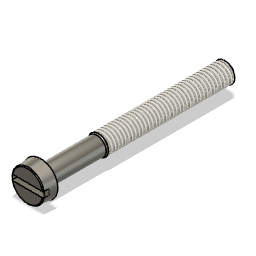
Drill_Jig_Assembly (Autodesk Fusion 360 archive; units mm, degrees)
design "Cheese Head Screw ISO 1207 - M6 x 55 Steel 10.9 Plain"
description: Cheese Head Screw ISO 1207 - M6 x 55
Autodesk Fusion 360 part; units mm, degrees
sketch "Sketch1" plane through (0, 0, 0) normal (0, 1, 0) x (1, 0, 0)
  line L0 (-3, 55) -> (0, 55)
  line L1 (0, 55) -> (0, -3.9)
  line L2 (-2.6932, 0) -> (-5, 0)
  line L3 (0, -3.9) -> (-4.4297, -3.9)
  line L4 (-4.6788, -3.6718) -> (-5, 0)
  arc A0 (-4.6788, -3.6718) -> (-4.4297, -3.9) centre (-4.4297, -3.65) ccw
  line L5 (-2.6932, 0) -> (-2.6932, 16.4687)
  line L6 (-3, 17) -> (-3, 55)
  line L7 (-3, 55) -> (0, 55)
  line L8 (-3, 17) -> (-2.6932, 16.4687)
  line L9 (0, -1.75) -> (0, -22.5)
  dimension "d66" = 10
  dimension "d67" = 3.9
  dimension "d68" = 55
  dimension "d83" = 0.25
  dimension "d93" = 5.3865
  dimension "d95" = 6
  dimension "d97" = 150
  dimension "d98" = 17
  dimension "d100" = 85
  constraint collinear origin L1.end L0.end
  constraint coincident origin L2
  constraint vertical L1
  constraint perpendicular L1 L3
  constraint tangent L3 A0
  constraint tangent L4 A0
  constraint perpendicular L2 L5
  constraint perpendicular L2 L6
  constraint perpendicular L6 L7
  constraint coincident L0.start L6.end
  measures "d67" vertical distance of L1.end L2.end
  measures "d68" distance of origin L0.end
  measures "d83" radius of A0
  measures "d97" angle of L6 L8
  measures "d98" vertical distance of L2.start L6.start
  measures "d100" angle of L2 L4
revolve "Revolve1" add sketch "Sketch1" angle 360 about axis through (0, 0, -55) along (0, 0, 1)
ref_plane "WorkPlane1" through (0, 0, 3.9) normal (0, 0, 1) x (1, 0, 0)
sketch "Sketch7" plane through (0, 0, 3.9) normal (0, 0, 1) x (1, 0, 0)
  line L0 (-4.6788, 0.8) -> (4.6788, 0.8)
  line L1 (4.6788, 0.8) -> (4.6788, -0.8)
  line L2 (4.6788, -0.8) -> (-4.6788, -0.8)
  line L3 (-4.6788, -0.8) -> (-4.6788, 0.8)
  line L4 (-4.6788, 0) -> (4.6788, 0) construction
  circle A0 centre (0, 0) radius 4.6788
  dimension "d77" = 1.6
  constraint horizontal L0
  constraint vertical L1
  constraint horizontal L2
  constraint vertical L3
  constraint midpoint L3 L4.start
  constraint midpoint L1 L4.end
  constraint coincident A0.centre L4
  constraint tangent L3 A0
  constraint tangent L1 A0
  measures "d77" distance of L0.end L1.end
extrude "Extrude3" cut sketch "Sketch7" against normal blind 1.6 contours L0 L2 A0
thread "Thread1" "ISO Metric profile 6.0 M6x1 6g" major diameter 5.884 minor diameter 4.7435 pitch 1 angle 60 resizes the face on face at (-2.9963, 0.1495, -29.6667)
sketch "Sketch8" plane through (0, 0, 0) normal (0, 1, 0) x (1, 0, 0)
  line L0 (0, 55) -> (0, -3.9)
  line L1 (0, 55) -> (-3.06, 55)
  line L2 (-3.06, 55) -> (-3.06, 53.8)
  line L3 (-3.06, 53.8) -> (-1.5, 55)
  dimension "d109" = 1.5
  dimension "d110" = 3.06
  dimension "d111" = 1.2
  constraint coincident L0.start L1.start
  constraint perpendicular L0 L1
  constraint perpendicular L1 L2
  constraint coincident L1 L3.end
  measures "d109" horizontal distance of origin L3.end
  measures "d110" horizontal distance of origin L1.end
  measures "d111" distance of L1.end L2.end
revolve "Revolve3" cut sketch "Sketch8" angle 360 about axis through (0, 0, 1.75) along (0, 0, 1)
equation "adsk_nomlen = 55.00 mm"
equation "adsk_headh = 3.90 mm"
equation "adsk_headdia = 10.00 mm"
equation "adsk_nomdia = 6.00 mm"
equation "d66 = adsk_headdia"
equation "d67 = adsk_headh"
equation "d68 = adsk_nomlen"
equation "d71 = adsk_headh"
equation "adsk_slotdepth = 1.60 mm"
equation "adsk_slotw = 1.60 mm"
equation "d77 = adsk_slotw"
equation "d78 = -adsk_slotdepth"
equation "adsk_thrlen = 38.00 mm"
equation "d83 = adsk_headr"
equation "adsk_headr = 0.25 mm"
equation "d93 = adsk_grpdia"
equation "d95 = adsk_nomdia"
equation "d98 = adsk_nomlen - adsk_thrlen"
equation "adsk_grpdia = 5.3865 mm"
equation "adsk_endpointdia = adsk_nomdia / 2"
equation "adsk_startlen = 0.2 * adsk_nomdia"
equation "d109 = adsk_endpointdia / 2"
equation "d110 = adsk_nomdia * 0.51"
equation "d111 = adsk_startlen"

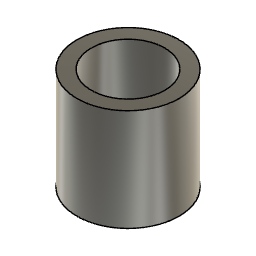
design "Bush case case hardened"
Autodesk Fusion 360 part; units mm, degrees
sketch "Sketch1" plane through (0, 0, 0) normal (0, 1, 0) x (1, 0, 0)
  line L0 (9, -12.5) -> (9, 0)
  line L1 (12.5, 0) -> (12.5, -12.5)
  line L2 (12.5, -12.5) -> (9, -12.5)
  line L3 (12.5, 0) -> (12.5, 12.5)
  line L4 (12.5, 12.5) -> (9, 12.5)
  line L5 (9, 12.5) -> (9, 0)
  line L6 (0, 0) -> (0, -12.5)
  line L7 (0, -12.5) -> (0, 12.5)
  dimension "d3" = 12.5
  constraint perpendicular L0 L2
  constraint coincident L6.start origin
  constraint perpendicular L2 L6
  constraint perpendicular L4 L7
  measures "d3" distance of L6.start L1.start
revolve "Revolve1" add sketch "Sketch1" angle 360 about axis through (0, 0, 12.5) along (0, 0, -1)
equation "d3 = ( 25 / 2 ) * 1 mm"

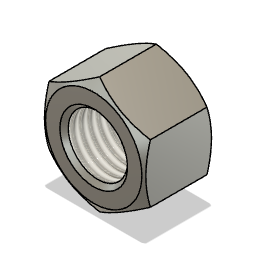
design "Hexagon High Nut ISO 4033 - M20 Steel 6 Plain"
description: Hexagon High Nut ISO 4033 - M20
Autodesk Fusion 360 part; units mm, degrees
sketch "Sketch1" plane through (0, 0, 0) normal (0, 1, 0) x (1, 0, 0)
  line L0 (0, 0.8114) -> (0, -2.1886)
  line L1 (-10, 0) -> (-14.25, 0)
  line L2 (-14.25, 0) -> (-17.325, -1.7754)
  line L3 (-17.325, -1.7754) -> (-17.325, -18.5246)
  line L4 (-17.325, -18.5246) -> (-14.25, -20.3)
  line L5 (-14.25, -20.3) -> (-10, -20.3)
  line L6 (-10, -20.3) -> (-10, 0)
  dimension "d121" = 20
  dimension "d122" = 30
  dimension "d123" = 30
  dimension "d125" = 28.5
  dimension "d126" = 20.3
  dimension "d127" = 28.5
  dimension "d128" = 34.65
  constraint vertical L0
  constraint coincident L0 L0.end
  constraint coincident origin L0
  constraint horizontal L1
  constraint perpendicular L1 L3
  constraint perpendicular L3 L5
  constraint perpendicular L5 L6
  constraint coincident origin L1
  measures "d122" angle of L1 L2
  measures "d123" angle of L4 L5
  measures "d126" distance of L1.start L5.end
revolve "Revolve1" add sketch "Sketch1" angle 360 about axis through (0, 0, -0.8114) along (0, 0, 1)
sketch "Sketch8" plane through (0, 0, 20.3) normal (0, 0, 1) x (1, 0, 0)
  line L0 (0, 0) -> (-30, 0) construction
  line L1 (-15, -8.6692) -> (-15, 8.6692)
  circle A0 centre (0, 0) radius 10
  circle A1 centre (0, 0) radius 17.325
  dimension "d114" = 15
  constraint horizontal L0
  constraint perpendicular L0 L1
  constraint midpoint L0 L1
  constraint coincident L0.start A0.centre
  constraint coincident L1.end A1
  measures "d114" distance of L0.start L1
extrude "Extrude5" cut sketch "Sketch8" against normal blind 20.3 contours L1 A1 picked at (-15.3751, 2.1116)
pattern_circular "C-Pattern2" count 6 over 360 about axis through (0, 0, 1.75) along (0, 0, 1) of "Extrude5"
thread "Thread3" "ISO Metric profile 20.0 M20x2.5 6H" major diameter 20.2925 minor diameter 17.519 pitch 2.5 angle 60 resizes the face on face at (-9.9503, 0.9957, 13.5333)
sketch "Sketch12" plane through (0, 0, 0) normal (0, 1, 0) x (1, 0, 0)
  line L0 (8.7595, -20.3) -> (-8.7595, -20.3)
  line L1 (14.25, -20.3) -> (-14.25, -20.3)
  line L2 (14.25, 0) -> (-14.25, 0)
  line L3 (8.7595, 0) -> (-8.7595, 0)
  line L4 (-10, 0) -> (-7, 0)
  line L5 (-7, 0) -> (-7, -3)
  line L6 (-7, -3) -> (-10, 0)
  line L7 (-10, -20.3) -> (-7, -20.3)
  line L8 (-7, -20.3) -> (-7, -17.3)
  line L9 (-7, -17.3) -> (-10, -20.3)
  line L10 (0, -1.75) -> (0, -22.5)
  dimension "d165" = 45
  dimension "d166" = 10
  dimension "d167" = 3
  dimension "d169" = 45
  constraint horizontal L4
  constraint perpendicular L4 L5
  constraint perpendicular L5 L7
  constraint perpendicular L2 L8
  constraint equal L5 L8
  constraint collinear L1 L7
  constraint collinear L2 L4
  constraint collinear L5 L8
  measures "d165" angle of L2 L6
  measures "d166" distance of L4.start L10
  measures "d167" distance of L4.end L5.end
  measures "d169" angle of L7 L9
revolve "Revolve3" cut sketch "Sketch12" angle 360 about axis through (0, 0, 1.75) along (0, 0, 1)
equation "adsk_nheig = 20.30 mm"
equation "adsk_maxdia = 34.65 mm"
equation "adsk_nomdia = 20.00 mm"
equation "d89 = -adsk_nheig"
equation "adsk_waflat = 30.00 mm"
equation "d114 = adsk_waflat / 2"
equation "adsk_chamang1 = 30.00 deg"
equation "adsk_chamang2 = 30.00 deg"
equation "d121 = adsk_nomdia"
equation "d122 = adsk_chamang1"
equation "d123 = adsk_chamang2"
equation "d125 = adsk_waflat * 0.95"
equation "d126 = adsk_nheig"
equation "d127 = adsk_waflat * 0.95"
equation "d128 = adsk_maxdia"
equation "d163 = adsk_nheig"
equation "d166 = adsk_nomdia * 0.5"
equation "d167 = adsk_nomdia * 0.15"

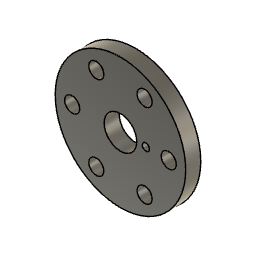
design "jig plate"
Autodesk Fusion 360 part; units mm, degrees
sketch "Sketch1" plane through (0, 0, 0) normal (0, 1, 0) x (1, 0, 0)
sketch "Sketch2" plane through (0, 0, 0) normal (0, 0, 1) x (1, 0, 0)
sketch "Sketch3" plane through (0, 0, 0) normal (0, 1, 0) x (1, 0, 0)
  circle A0 centre (0, 0) radius 108
  dimension "d1" = 216
  constraint coincident A0.centre origin
  measures "d1" diameter of A0
extrude "Extrude1" add sketch "Sketch3" along normal blind 25
sketch "Sketch4" plane through (0, 25, 0) normal (0, 1, 0) x (-1, 0, 0)
  circle A0 centre (0, 0) radius 108
  circle A1 centre (0, 0) radius 27
  line L0 (0, 0) -> (-80, 0)
  circle A2 centre (-80, 0) radius 12.5
  circle A3 centre (0, 0) radius 80
  dimension "d4" = 54
  dimension "d7" = 80
  dimension "d8" = 25
  constraint concentric A0 A1
  constraint coincident A0.centre A1.centre
  constraint horizontal L0
  constraint coincident L0.end A2.centre
  constraint concentric A0 A3
  constraint coincident L0.end A3
  measures "d4" diameter of A1
  measures "d7" distance of A0.centre L0.end
  measures "d8" diameter of A2
extrude "Extrude2" cut sketch "Sketch4" against normal blind 200 contours A1
sketch "Sketch5" plane through (0, 25, 0) normal (0, 1, 0) x (-1, 0, 0)
  circle A0 centre (0, 0) radius 27
  circle A1 centre (0, 0) radius 108
  circle A2 centre (-80, 0) radius 12.5
  circle A3 centre (-40, -69.282) radius 12.5
  circle A4 centre (40, -69.282) radius 12.5
  circle A5 centre (80, 0) radius 12.5
  circle A6 centre (40, 69.282) radius 12.5
  circle A7 centre (-40, 69.282) radius 12.5
  dimension "d9" = 80
  dimension "d10" = 25
  measures "d9" distance of A0.centre A2.centre
  measures "d10" diameter of A2
extrude "Extrude3" cut sketch "Sketch5" against normal blind 200 contours A2 | A3 | A4 | A5 | A6 | A7
sketch "Sketch6" plane through (0, 25, 0) normal (0, 1, 0) x (-1, 0, 0)
  circle A0 centre (-40, -69.282) radius 12.5
  circle A1 centre (40, 69.282) radius 12.5
  circle A2 centre (-80, 0) radius 12.5
  circle A3 centre (40, -69.282) radius 12.5
  circle A4 centre (80, 0) radius 12.5
  circle A5 centre (-40, 69.282) radius 12.5
  circle A6 centre (0, 0) radius 27
  circle A7 centre (0, 0) radius 108
  line L0 (0, 0) -> (-42, 0)
  circle A8 centre (-42, 0) radius 8.5
  dimension "d15" = 42
  dimension "d16" = 17
  constraint coincident A6.centre A7.centre
  constraint horizontal L0
  constraint coincident L0.end A8.centre
  measures "d15" distance of A6.centre L0.end
  measures "d16" diameter of A8
extrude "Extrude4" cut sketch "Sketch6" against normal blind 9 contours A8
sketch "Sketch7" plane through (0, 16, 0) normal (0, 1, 0) x (-1, 0, 0)
  circle A0 centre (-42, 0) radius 8.5
  circle A1 centre (-42, 0) radius 6
  dimension "d19" = 12
  constraint concentric A0 A1
  measures "d19" diameter of A1
extrude "Extrude5" cut sketch "Sketch7" against normal blind 100 contours A1

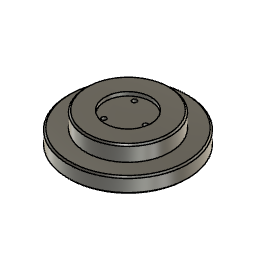
design "base plate"
Autodesk Fusion 360 part; units mm, degrees
sketch "Sketch1" plane through (0, 0, 0) normal (0, 1, 0) x (1, 0, 0)
  line L0 (0, 0) -> (0, -15)
  line L1 (0, 0) -> (0, 20)
  line L2 (0, 20) -> (76, 20)
  line L3 (78, 18) -> (78, 2)
  line L4 (30, -20) -> (30, -15)
  line L5 (30, -15) -> (0, -15)
  line L6 (55, -18) -> (55, 0)
  line L7 (55, 0) -> (76, 0)
  line L8 (20, -15) -> (26, -15)
  line L9 (30, -20) -> (53, -20)
  line L10 (55, -18) -> (53, -20)
  line L11 (78, 2) -> (76, 0)
  line L12 (76, 20) -> (78, 18)
  point P0 (78, 20)
  point P1 (78, 0)
  point P2 (55, -20)
  dimension "d2" = 20
  dimension "d3" = 78
  dimension "d4" = 20
  dimension "d6" = 5
  dimension "d8" = 6
  dimension "d10" = 2
  dimension "d11" = 2
  dimension "d12" = 2
  dimension "d13" = 2
  dimension "d14" = 2
  dimension "d15" = 2
  constraint coincident L0.start L1.start
  constraint vertical L0
  constraint parallel L0 L1
  constraint perpendicular L1 L2
  constraint perpendicular L2 L3
  constraint perpendicular L0 L5
  constraint perpendicular L3 L7
  constraint coincident L5 L8.start
  constraint coincident P2 L6
  constraint coincident P2 L9
  constraint coincident P1 L3
  constraint coincident P1 L7
  constraint coincident P0 L2
  constraint coincident P0 L3
  measures "d2" distance of L0.start L1.end
  measures "d3" distance of L1.end P0
  measures "d4" distance of P0 P1
  measures "d6" distance of L4.start L4.end
  measures "d8" distance of L8.start L8.end
  measures "d10" distance of P2 L6.start
  measures "d11" distance of P2 L9.end
  measures "d12" distance of P1 L3.end
  measures "d13" distance of P1 L7.end
  measures "d14" distance of P0 L2.end
  measures "d15" distance of P0 L3.start
revolve "Revolve1" add sketch "Sketch1" angle 360 about axis through (0, 0, 0) along (0, 0, 1)
sketch "Sketch2" plane through (0, 0, -20) normal (0, 0, -1) x (1, 0, 0)
  circle A0 centre (0, 0) radius 76
  circle A1 centre (23, 0) radius 3
  dimension "d17" = 23
  dimension "d18" = 6
  measures "d17" distance of A0.centre A1.centre
  measures "d18" diameter of A1
extrude "Extrude1" cut sketch "Sketch2" against normal blind 300 contours A1
sketch "Sketch3" plane through (0, 0, -20) normal (0, 0, -1) x (1, 0, 0)
  circle A0 centre (23, 0) radius 3
  circle A1 centre (0, 0) radius 76
  circle A2 centre (23, 0) radius 4
  dimension "d21" = 8
  constraint concentric A0 A2
  measures "d21" diameter of A2
extrude "Extrude2" cut sketch "Sketch3" against normal blind 8 contours A2
sketch "Sketch4" plane through (0, 0, -20) normal (0, 0, -1) x (1, 0, 0)
  circle A0 centre (23, 0) radius 4
  circle A1 centre (0, 0) radius 76
  circle A2 centre (-11.5, 19.9186) radius 4
  circle A3 centre (-11.5, -19.9186) radius 4
  dimension "d25" = 360
extrude "Extrude3" cut sketch "Sketch4" against normal blind 8 contours A2 | A3
sketch "Sketch5" plane through (0, 0, -12) normal (0, 0, -1) x (1, 0, 0)
  circle A0 centre (-11.5, 19.9186) radius 4
  circle A1 centre (-11.5, 19.9186) radius 3
  dimension "d28" = 6
  constraint concentric A0 A1
  measures "d28" diameter of A1
extrude "Extrude4" cut sketch "Sketch5" against normal blind 200 contours A1
sketch "Sketch6" plane through (0, 0, -12) normal (0, 0, -1) x (1, 0, 0)
  circle A0 centre (-11.5, -19.9186) radius 4
  circle A1 centre (-11.5, -19.9186) radius 3
  dimension "d31" = 6
  constraint concentric A0 A1
  measures "d31" diameter of A1
extrude "Extrude5" cut sketch "Sketch6" against normal blind 300 contours A1
equation "d3 = ( 156 / 2 ) * 1 mm"
equation "d11 = d10"
equation "d13 = d12"
equation "d15 = d14"

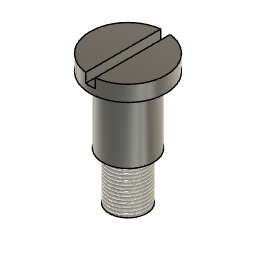
design "screw"
Autodesk Fusion 360 part; units mm, degrees
sketch "Sketch1" plane through (0, 0, 0) normal (0, 1, 0) x (1, 0, 0)
  line L0 (0, 0) -> (0, -15)
  line L1 (0, 0) -> (6, 0)
  line L2 (6, 0) -> (6, -15)
  line L3 (0, 0) -> (0, -36)
  line L4 (8, -36) -> (8, -15)
  line L5 (8, -15) -> (6, -15)
  line L6 (8, -36) -> (12, -36)
  line L7 (12, -36) -> (12, -41)
  line L8 (12, -41) -> (0, -41)
  line L9 (0, -41) -> (0, -36)
  dimension "d1" = 15
  dimension "d2" = 6
  dimension "d3" = 36
  dimension "d4" = 8
  dimension "d5" = 12
  dimension "d6" = 5
  constraint coincident L0.start L1.start
  constraint vertical L0
  constraint perpendicular L0 L1
  constraint perpendicular L1 L2
  constraint perpendicular L1 L3
  constraint perpendicular L2 L5
  constraint perpendicular L3 L6
  constraint perpendicular L6 L7
  constraint perpendicular L3 L8
  constraint perpendicular L6 L9
  measures "d1" distance of L0.start L0.end
  measures "d2" distance of L0.start L1.end
  measures "d3" distance of L0.start L3.end
  measures "d4" distance of L3.end L4.start
  measures "d5" distance of L3.end L6.end
  measures "d6" distance of L6.end L7.end
revolve "Revolve1" add sketch "Sketch1" angle 360 about axis through (0, 0, 0) along (0, 0, 1)
sketch "Sketch2" plane through (0, 0, 41) normal (0, 0, 1) x (-1, 0, 0)
  circle A0 centre (0, 0) radius 12
  line L0 (1.5, -11.9059) -> (1.5, 11.9059)
  line L1 (-1.5, 11.9059) -> (-1.5, -11.9059)
  line L2 (-0.9084, -11.9656) -> (0.9084, 11.9656) construction
  line L3 (0.9084, -11.9656) -> (-0.9084, 11.9656) construction
  constraint parallel L0 L1
  constraint coincident L2 A0.centre
  constraint coincident L3 A0.centre
  constraint coincident A0.centre origin
  constraint coincident A0 L1.end
  constraint coincident A0 L2.start
  constraint coincident A0 L3.start
  constraint coincident A0 L0.start
  constraint coincident A0 L1.start
  constraint coincident A0 L3.end
  constraint coincident A0 L2.end
  constraint coincident A0 L0.end
extrude "Extrude1" cut sketch "Sketch2" against normal blind 3 contours A0 L0 L1
thread "Thread1" "ISO Metric profile 12.0 M12x1 6g" major diameter 11.884 minor diameter 10.7405 pitch 1 angle 60 resizes the face on face at (5.9702, -0.5974, 10) from (0, 0, 0) to (0, 0, 15)

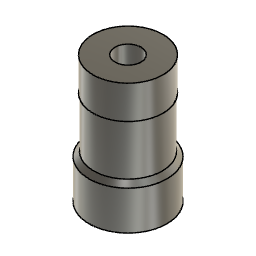
design "stem"
Autodesk Fusion 360 part; units mm, degrees
sketch "Sketch1" plane through (0, 0, 0) normal (0, 1, 0) x (1, 0, 0)
  line L0 (0, 0) -> (30, 0)
  line L1 (0, 0) -> (0, -44)
  line L2 (10, -98) -> (27, -98)
  line L3 (27, -98) -> (27, -72.3867)
  line L4 (30, 0) -> (30, -25)
  line L5 (30, -25) -> (30, -30)
  line L6 (30, -30) -> (26.4645, -33.5355)
  line L7 (26.4645, -33.5355) -> (26.4645, -72.3867)
  line L8 (26.4645, -72.3867) -> (27, -72.3867)
  line L9 (10, -98) -> (10, -44)
  line L10 (10, -44) -> (0, -44)
  dimension "d1" = 30
  dimension "d5" = 25
  dimension "d6" = 5
  dimension "d7" = 5
  dimension "d9" = 54
  constraint coincident L0.start L1.start
  constraint horizontal L0
  constraint vertical L1
  constraint perpendicular L1 L2
  constraint perpendicular L2 L3
  constraint perpendicular L0 L4
  constraint parallel L4 L5
  constraint parallel L3 L7
  constraint perpendicular L3 L8
  constraint perpendicular L2 L9
  constraint perpendicular L1 L10
  measures "d1" distance of L0.start L0.end
  measures "d5" distance of L0.end L4.end
  measures "d6" distance of L4.end L5.end
  measures "d7" distance of L5.end L6.end
  measures "d9" distance of L2.start L9.end
revolve "Revolve1" add sketch "Sketch1" angle 360 about axis through (0, 0, 0) along (0, 0, 1)
sketch "Sketch2" plane through (0, 0, 0) normal (0, 0, -1) x (1, 0, 0)
  circle A0 centre (0, 0) radius 30
  circle A1 centre (20, 0) radius 3
  circle A2 centre (-10, 17.3205) radius 3
  circle A3 centre (-10, -17.3205) radius 3
  dimension "d12" = 6
  measures "d12" diameter of A1

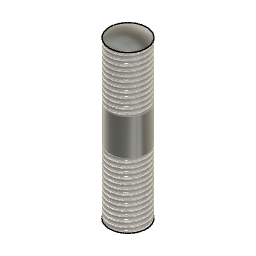
design "STUD 2"
Autodesk Fusion 360 part; units mm, degrees
sketch "Sketch1" plane through (0, 0, 0) normal (0, 1, 0) x (1, 0, 0)
  line L0 (10, -42) -> (0, -42)
  line L1 (0, 42) -> (10, 42)
  line L2 (10, 42) -> (10, -42)
  arc A0 (10, 42) -> (0, 45) centre (0, 26.8333) ccw
  arc A1 (0, -45) -> (10, -42) centre (0, -26.8333) ccw
  line L3 (0, -45) -> (0, 45)
  line L4 (0, 45) -> (0, -45)
  constraint horizontal L0
  constraint parallel L0 L1
  constraint perpendicular L0 L4
  constraint coincident L3 L0.end
  constraint coincident L3 L1.start
revolve "Revolve1" add sketch "Sketch1" angle 360 about axis through (0, 0, -45) along (0, 0, 1)
thread "Thread1" "ISO Metric profile 20.0 M20x2.5 6g" major diameter 19.7905 minor diameter 16.938 pitch 2.5 angle 60 resizes the face on face at (9.9503, -0.9957, 14) from (0, 0, -42) to (0, 0, -7)
thread "Thread2" "ISO Metric profile 20.0 M20x2.5 6g" major diameter 19.7905 minor diameter 16.938 pitch 2.5 angle 60 resizes the face on face at (9.8847, 0.4579, -14.0228) from (0, 0, 12.0685) to (0, 0, 42.0685)

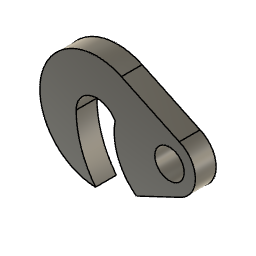
design "latch washer"
Autodesk Fusion 360 part; units mm, degrees
sketch "Sketch1" plane through (0, 0, 0) normal (0, 1, 0) x (1, 0, 0)
  circle A0 centre (42, 0) radius 8.5
  arc A1 (-0.75, 32.9915) -> (-12, 0) centre (42, 0) ccw
  arc A2 (-0.75, 32.9915) -> (14.1623, -29.8065) centre (0, 0) ccw
  line L0 (47.6493, -13.8955) -> (14.1623, -29.8065)
  arc A3 (22.8838, 25.6626) -> (10.5238, -5.7662) centre (42, 0) ccw
  arc A4 (-12, 0) -> (10.5238, -5.7662) centre (0, 0) ccw
  line L1 (47.6493, 13.8955) -> (22.8838, 25.6626)
  arc A5 (47.6493, -13.8955) -> (47.6493, 13.8955) centre (42, 0) ccw
  arc A6 (47.6493, -13.8955) -> (47.6493, 13.8955) centre (42, 0) ccw
  dimension "d1" = 66
  dimension "d2" = 42
  dimension "d3" = 17
  dimension "d4" = 30
  dimension "d5" = 108
  dimension "d6" = 24
  dimension "d7" = 64
  constraint coincident A2.centre A4.centre
  constraint concentric A0 A5
  constraint concentric A0 A1
  constraint concentric A2 A4
  constraint concentric A1 A3
  constraint tangent A2 L0
  measures "d1" diameter of A2
  measures "d2" distance of A2.centre A0.centre
  measures "d3" diameter of A0
  measures "d4" diameter of A5
  measures "d5" diameter of A1
  measures "d6" diameter of A4
  measures "d7" diameter of A3
extrude "Extrude1" add sketch "Sketch1" along normal blind 12
equation "d5 = 54 mm + 54 mm"
